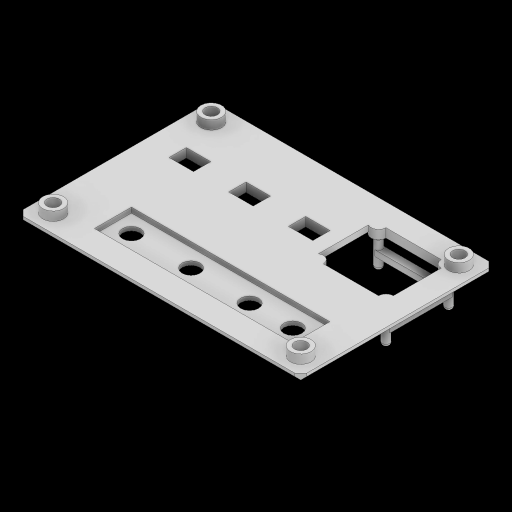
# Autodesk Inventor part: gora
Saved by Autodesk Inventor 2024.4 (Build 284460000, 460)
## iProperties
Created: 2026-01-14
Part Number: gora
Material: Ogólny
Document SubType Name: Modeling
Designer: User
Density: 1 g/cm^3
Appearance: Domyślna
Author: User
Autodesk Inventor part; units mm, degrees
ref_plane "YZ Plane" through (0, 0, 0) normal (1, 0, 0) x (0, 1, 0)
ref_plane "XZ Plane" through (0, 0, 0) normal (0, 1, 0) x (-1, 0, 0)
ref_plane "XY Plane" through (0, 0, 0) normal (0, 0, 1) x (1, 0, 0)
sketch "Szkic1" plane through (0, 0, 0) normal (0, 1, 0) x (-1, 0, 0)
  line L0 (-47.5, 32.5) -> (47.5, 32.5)
  line L1 (47.5, 32.5) -> (47.5, -32.5)
  line L2 (47.5, -32.5) -> (-47.5, -32.5)
  line L3 (-47.5, -32.5) -> (-47.5, 32.5)
  line L4 (-47.5, 32.5) -> (47.5, -32.5) construction
  line L5 (47.5, 32.5) -> (-47.5, -32.5) construction
  point P0 (0, 0)
  dimension "d0" = 95
  dimension "d1" = 65
  constraints: 12 end point, 2 midpoint, 2 parallel, 1 horizontal, 1 perpendicular
  measures "d0" distance of L1.end L2.end
  measures "d1" distance of L0.end L1.end
extrude "Wyciągnięcie proste1" add sketch "Szkic1" along normal blind 3
chamfer "Faza1" distance 2 angle 45 4 edges at (47.5, 1.5, 32.5) (47.5, 1.5, -32.5) (-47.5, 1.5, 32.5) (-47.5, 1.5, -32.5)
sketch "Szkic4" plane through (0, 0, 0) normal (0, -1, 0) x (1, 0, 0)
  line L0 (41.8196, -27.3452) -> (14.8196, -27.3452)
  line L1 (16.8196, -2.3452) -> (41.8196, -2.3452)
  line L2 (15.8196, -27.5) -> (42.8196, -27.5)
  line L3 (41.8196, -2.3452) -> (41.8196, -27.3452)
  line L4 (41.8196, -27.3452) -> (14.8196, -2.3452) construction
  line L5 (14.8196, -27.3452) -> (41.8196, -2.3452) construction
  circle A0 centre (39.5696, -25) radius 1.25
  circle A1 centre (38.3196, -4.5952) radius 1.25
  circle A2 centre (39.5696, -4) radius 1.25
  circle A3 centre (17.3196, -4.5952) radius 1.25
  circle A4 centre (16.0696, -4) radius 1.25
  circle A5 centre (17.3196, -28.0952) radius 1.25
  circle A6 centre (16.0696, -25) radius 1.25
  circle A7 centre (38.3196, -28.0952) radius 1.25
  line L6 (13.8196, -2.3452) -> (13.8196, -28.3452)
  line L7 (12.8196, -1.5) -> (40.8196, -1.5)
  line L8 (41.8196, -28.3452) -> (41.8196, -2.3452)
  line L9 (14.8196, -2.3452) -> (14.8196, -30.3452)
  line L10 (14.8196, -30.3452) -> (40.8196, -2.3452) construction
  line L11 (40.8196, -30.3452) -> (14.8196, -2.3452) construction
  line L12 (34.7997, -21.2897) -> (22.7997, -21.2897)
  line L13 (22.7997, -21.2897) -> (22.7997, -9.2897)
  line L14 (22.7997, -9.2897) -> (34.7997, -9.2897)
  line L15 (34.7997, -9.2897) -> (34.7997, -21.2897)
  line L16 (34.7997, -21.2897) -> (22.7997, -9.2897) construction
  line L17 (22.7997, -21.2897) -> (34.7997, -9.2897) construction
  line L18 (39.5696, -25) -> (16.0696, -25)
  line L19 (16.0696, -25) -> (16.0696, -4)
  line L20 (16.0696, -4) -> (39.5696, -4)
  line L21 (39.5696, -4) -> (39.5696, -25)
  circle A8 centre (16.0696, -25) radius 2.5
  circle A9 centre (39.5696, -25) radius 2.5
  circle A10 centre (39.5696, -4) radius 2.5
  circle A11 centre (16.0696, -4) radius 2.5
  line L22 (45.5, -32.5) -> (-45.5, -32.5) projected
  point P0 (0, 0)
  point P1 (28.3196, -14.8452)
  point P2 (27.8196, -16.3452)
  point P3 (28.7997, -15.2897)
  point P4 (18.5696, -4)
  point P5 (16.0696, -6.5)
  point P6 (16.0696, -22.5)
  point P7 (18.5696, -25)
  point P8 (37.0696, -25)
  point P9 (39.5696, -22.5)
  point P10 (39.5696, -6.5)
  point P11 (37.0696, -4)
  dimension "d36" = 27
  dimension "d37" = 25
  dimension "d41" = 26
  dimension "d42" = 28
  dimension "d43" = 12
  dimension "d44" = 12
  dimension "d62" = 18.5
  dimension "d63" = 5
  dimension "d64" = 5
  dimension "d65" = 5
  dimension "d66" = 5
  dimension "d79" = 7.5
  dimension "d80" = 2.5
  dimension "d81" = 90
  dimension "d82" = 42.797
  dimension "d83" = 137.203
  dimension "d84" = 132.879
  dimension "d85" = 47.121
  dimension "d86" = 90
  dimension "d87" = 5.1548
  dimension "d88" = 23.2103
  dimension "d89" = 28
  dimension "d90" = 4.7699
  dimension "d91" = 23.5
  dimension "d92" = 3.6804
  dimension "d93" = 3.6804
  dimension "d94" = 30.1548
  dimension "d95" = 24.6269
  dimension "d96" = 1.9635
  dimension "d97" = 30.1548
  dimension "d98" = 30.1548
  dimension "d99" = 30.1548
  dimension "d100" = 30.1548
  dimension "d101" = 2.1548
  dimension "d102" = 25.1548
  dimension "d103" = 9.1548
  dimension "d104" = 27.9048
  dimension "d105" = 4.4048
  dimension "d106" = 27.6548
  dimension "d107" = 6.6548
  dimension "d108" = 27.6548
  dimension "d109" = 6.6548
  dimension "d110" = 27.9048
  dimension "d111" = 4.4048
  dimension "d112" = 25.1548
  dimension "d113" = 9.1548
  dimension "d114" = 30.1548
  dimension "d115" = 2.1548
  dimension "d116" = 30.1548
  dimension "d117" = 4.1548
  dimension "d118" = 1
  dimension "d119" = 0
  dimension "d120" = 1
  dimension "d121" = 2.25
  dimension "d122" = 2.25
  dimension "d123" = 4.75
  dimension "d124" = 4.75
  dimension "d125" = 23.25
  dimension "d126" = 23.25
  dimension "d127" = 25.75
  dimension "d128" = 25.75
  dimension "d129" = 27
  constraints: 44 end point, 12 centre point, 9 tangent, 7 parallel, 6 equal radius, 6 midpoint, 4 coincident, 3 horizontal, 3 perpendicular, 2 concentric, 2 point on line
  measures "d36" distance of L2.start L2.end
  measures "d37" distance of L1.start L1.end
  measures "d41" distance of L8.end L8.start
  measures "d42" distance of L7.start L7.end
  measures "d43" distance of L13.end L14.end
  measures "d44" distance of L12.end L13.end
  measures "d63" diameter of A8
  measures "d64" diameter of A9
  measures "d65" diameter of A10
  measures "d66" diameter of A11
  measures "d79" distance between parallel lines of L22 L18
  measures "d80" diameter of A2
  measures "d81" angle of L3 L22
  measures "d82" angle of L4 L22
  measures "d83" angle of L5 L22
  measures "d84" angle of L10 L22
  measures "d85" angle of L11 L22
  measures "d86" angle of L3 L1
  measures "d87" distance between parallel lines of L0 L22
  measures "d88" distance between parallel lines of L14 L22
  measures "d89" distance between parallel lines of L8 L6
  measures "d90" distance between parallel lines of L21 L15
  measures "d91" distance between parallel lines of L21 L19
  measures "d92" distance from line of L22.start L3
  measures "d93" distance from line of L22.start L8
  measures "d94" distance from line of L22.start L1
  measures "d95" distance from line of L22.start L5
  measures "d96" distance from line of L22.start L11
  measures "d97" distance from line of L8.end L22
  measures "d98" distance from line of L3.start L22
  measures "d99" distance from line of L5.end L22
  measures "d100" distance from line of L10.end L22
  measures "d101" distance from line of L11.start L22
  measures "d104" distance from line of A1.centre L22
  measures "d105" distance from line of A7.centre L22
  measures "d110" distance from line of A3.centre L22
  measures "d111" distance from line of A5.centre L22
  measures "d114" distance from line of L9.start L22
  measures "d115" distance from line of L9.end L22
  measures "d116" distance from line of L6.start L22
  measures "d117" distance from line of L6.end L22
  measures "d118" distance from line of L2.end L3
  measures "d119" distance from line of L1.end L3
  measures "d120" distance from line of L7.end L3
  measures "d121" distance from line of point (39.57, -6.5) L3
  measures "d122" distance from line of point (39.57, -22.5) L3
  measures "d123" distance from line of point (37.07, -4) L3
  measures "d124" distance from line of point (37.07, -25) L3
  measures "d125" distance from line of point (18.57, -4) L3
  measures "d126" distance from line of point (18.57, -25) L3
  measures "d127" distance from line of point (16.07, -6.5) L3
  measures "d128" distance from line of point (16.07, -22.5) L3
  measures "d129" distance from line of L0.end L3
extrude "Wyciągnięcie proste6" add sketch "Szkic4" along normal blind 10 contours L21 L18 A0 | A0 L18 L21 | L21 L20 A1 A2 | A2 A1 L21 | L18 L19 A6 | A6 L19 L18 | A2 L20 A1 | A1 L20 L21 | A2 A1 L20 | L19 A3 A4 | A4 A3 L20 L19 | A3 L20 A4 | L19 L20 A3 | A4 L20 A3 picked at (38.7441, -4.2892) picked at (38.9967, -3.9208) picked at (16.8951, -4.2892) picked at (16.6425, -3.9208)
fillet "Zaokrąglenie1" radius 1 4 edges at (14.8196, 0, -4) (14.8196, 0, -25) (38.3196, 0, -25) (38.3196, 0, -4)
sketch "Szkic6" plane through (0, 3, 0) normal (0, 1, 0) x (1, 0, 0)
  line L0 (47.5, -30.5) -> (47.5, 30.5) projected
  line L1 (47.5, 0) -> (-47.5, 0)
  line L2 (-47.5, 30.5) -> (-47.5, -30.5) projected
  line L3 (45.5, 32.5) -> (-45.5, 32.5) projected
  line L4 (0, 32.5) -> (0, -32.5)
  line L5 (-45.5, -32.5) -> (45.5, -32.5) projected
  circle A0 centre (41.5, -26.5) radius 2.1
  circle A1 centre (41.5, -26.5) radius 3.5
  line L6 (41.5, -26.5) -> (41.5, 26.5)
  circle A2 centre (41.5, 26.5) radius 2
  line L7 (41.5, -26.5) -> (-41.5, -26.5)
  line L8 (41.5, -26.5) -> (124.5, -26.5) construction
  circle A3 centre (-41.5, -26.5) radius 2
  point P0 (0, 0)
  dimension "d56" = 6
  dimension "d57" = 6
  dimension "d58" = 7
  dimension "d59" = 4.2
  dimension "d133" = 53
  dimension "d134" = 4
  dimension "d135" = 6
  dimension "d136" = 6
  dimension "d137" = 83
  dimension "d138" = 180
  dimension "d139" = 4
  dimension "d140" = 6
  dimension "d141" = 6
  constraints: 10 end point, 4 centre point, 4 midpoint, 3 coincident, 2 horizontal, 1 collinear, 1 vertical
  measures "d56" distance from line of L0 A0.centre
  measures "d57" distance from line of L5 A0.centre
  measures "d58" diameter of A1
  measures "d59" diameter of A0
  measures "d133" distance of L6.start L6.end
  measures "d134" diameter of A2
  measures "d135" distance from line of L3 A2.centre
  measures "d136" distance from line of L0 A2.centre
  measures "d137" distance of L6.start L7.end
  measures "d138" angle of L7 L8
  measures "d139" diameter of A3
  measures "d140" distance from line of L2 A3.centre
  measures "d141" distance from line of L5 A3.centre
extrude "Wyciągnięcie proste8" add sketch "Szkic6" along normal blind 3 contours L6 A0 L7 A1 | A1 L7 A0 L6
extrude "Wyciągnięcie proste9" cut sketch "Szkic4" against normal blind 4 contours A9 L18 A8 L19 A11 A3 L20 A10 A1 L21 | A1 A10 | A11 A3 | L12 L13 L14 L15
move faces "Przesuń3" translate (-1.25, 0, 0) faces at (16.0696, 1, -11.8333)
ref_plane "Płaszczyzna konstrukcyjna1" through (16.0696, -5, -4) normal (0, -1, 0) x (1, 0, 0)
sketch "Szkic7" plane through (16.0696, -5, -4) normal (0, -1, 0) x (1, 0, 0)
  circle A0 centre (0, 0) radius 1.25 projected
  circle A1 centre (23.5, 0) radius 1.25 projected
  line L0 (0, 1.25) -> (23.5, 1.25)
  line L1 (23.5, 1.25) -> (23.5, -1.25)
  line L2 (23.5, -1.25) -> (0, -1.25)
  line L3 (0, -1.25) -> (0, 1.25)
  circle A2 centre (23.5, -21) radius 1.25 projected
  line L4 (24.75, 0) -> (22.25, 0)
  line L5 (22.25, 0) -> (22.25, -21)
  line L6 (22.25, -21) -> (24.75, -21)
  line L7 (24.75, -21) -> (24.75, 0)
  line L8 (23.5, -22.25) -> (0, -22.25)
  line L9 (0, -22.25) -> (0, -19.75)
  line L10 (0, -19.75) -> (23.5, -19.75)
  line L11 (23.5, -19.75) -> (23.5, -22.25)
  circle A3 centre (0, -21) radius 1.25 projected
  line L12 (-1.25, -21) -> (1.25, -21)
  line L13 (1.25, -21) -> (1.25, 0)
  line L14 (1.25, 0) -> (-1.25, 0)
  line L15 (-1.25, 0) -> (-1.25, -21)
  point P0 (-16.0696, 4)
  point P1 (24.75, -21)
  point P2 (22.25, -1.25)
  point P3 (22.25, -19.75)
  point P4 (1.25, -19.75)
  point P5 (1.25, -1.25)
  constraints: 32 end point, 8 parallel, 7 point on circle, 4 horizontal, 4 perpendicular
extrude "Wyciągnięcie proste10" add sketch "Szkic7" along normal mid plane 2 contours L13 L2 A0 | A0 L0 A1 L5 L2 L13 | L2 A1 L7 A2 L10 L5 | L13 A3 L10 | L10 L5 A2 L8 A3 L13
fillet "Zaokrąglenie2" radius 1 4 edges at (14.8196, -10, -4) (14.8196, -10, -25) (38.3196, -10, -25) (38.3196, -10, -4)
chamfer "Faza2" distance 1 angle 45 1 edges at (14.8196, 0, -14.5)
mirror "Odbij1" about plane through (0, 0, 0) normal (0, 0, 1) of "Wyciągnięcie proste8"
mirror "Odbij2" about plane through (0, 0, 0) normal (1, 0, 0) of "Wyciągnięcie proste8", "Odbij1"
chamfer "Faza3" distance 2 angle 45 4 edges at (0, 0, -32.5) (47.5, 0, 0) (0, 0, 32.5) (-47.5, 0, 0)
sketch "Szkic8" plane through (0, 0, 0) normal (0, -1, 0) x (1, 0, 0)
  point P0 (0, 0)
sketch "Szkic9" plane through (0, 0, 0) normal (0, -1, 0) x (1, 0, 0)
  line L0 (-23.3666, -57.3233) -> (-23.3666, -67.3233)
  line L1 (-23.3666, -67.3233) -> (-33.3666, -67.3233)
  line L2 (-33.3666, -67.3233) -> (-33.3666, -57.3233)
  line L3 (-33.3666, -57.3233) -> (-23.3666, -57.3233)
  circle A0 centre (-28.3666, -62.3233) radius 1.65
  line L4 (-23.3666, -57.3233) -> (-33.3666, -67.3233) construction
  line L5 (-23.3666, -67.3233) -> (-33.3666, -57.3233) construction
  line L6 (-33.3666, -67.3233) -> (-33.3666, -57.3233)
  line L7 (-33.3666, -57.3233) -> (30.5704, -57.3233)
  line L8 (30.5704, -57.3233) -> (30.5704, -67.3233)
  line L9 (30.5704, -67.3233) -> (-33.3666, -67.3233)
  line L10 (-28.3666, -62.3233) -> (-28.3666, -82.3233)
  line L11 (-24.7466, -85.2233) -> (-24.7466, -79.6233)
  line L12 (-24.7466, -79.6233) -> (-31.1466, -79.6233)
  line L13 (-31.1466, -79.6233) -> (-31.1466, -85.2233)
  line L14 (-31.1466, -85.2233) -> (-24.7466, -85.2233)
  line L15 (-24.7466, -85.2233) -> (-31.1466, -79.6233) construction
  line L16 (-24.7466, -79.6233) -> (-31.1466, -85.2233) construction
  line L17 (-4.7466, -79.6233) -> (-11.1466, -79.6233)
  line L18 (-8.3666, -62.3233) -> (-8.3666, -82.3233)
  line L19 (-4.7466, -85.2233) -> (-4.7466, -79.6233)
  line L20 (-11.1466, -79.6233) -> (-11.1466, -85.2233)
  line L21 (-11.1466, -85.2233) -> (-4.7466, -85.2233)
  line L22 (-4.7466, -79.6233) -> (-11.1466, -85.2233) construction
  line L23 (-4.7466, -85.2233) -> (-11.1466, -79.6233) construction
  line L24 (15.2534, -79.6233) -> (8.8534, -79.6233)
  line L25 (11.6334, -62.3233) -> (11.6334, -82.3233)
  line L26 (15.2534, -85.2233) -> (15.2534, -79.6233)
  line L27 (8.8534, -79.6233) -> (8.8534, -85.2233)
  line L28 (8.8534, -85.2233) -> (15.2534, -85.2233)
  line L29 (15.2534, -79.6233) -> (8.8534, -85.2233) construction
  line L30 (15.2534, -85.2233) -> (8.8534, -79.6233) construction
  line L31 (-45.5, 30.5) -> (45.5, 30.5) projected
  line L32 (0, 30.5) -> (0, 17.7)
  line L33 (30.5, 20.7) -> (-30.5, 20.7)
  line L34 (-30.5, 20.7) -> (-30.5, 14.7)
  line L35 (-30.5, 14.7) -> (30.5, 14.7)
  line L36 (30.5, 14.7) -> (30.5, 20.7)
  line L37 (30.5, 20.7) -> (-30.5, 14.7) construction
  line L38 (-30.5, 20.7) -> (30.5, 14.7) construction
  line L39 (-30.5, 17.7) -> (-24.05, 17.7)
  circle A1 centre (-24.05, 17.7) radius 3
  circle A2 centre (-4.05, 17.7) radius 3
  circle A3 centre (15.95, 17.7) radius 3
  circle A4 centre (30.45, 17.7) radius 3
  point P0 (0, 0)
  point P1 (73.1005, -3.8431)
  point P2 (-27.9466, -82.4233)
  point P3 (-7.9466, -82.4233)
  point P4 (12.0534, -82.4233)
  dimension "d146" = 10
  dimension "d147" = 10
  dimension "d148" = 10
  dimension "d149" = 20
  dimension "d150" = 5.6
  dimension "d151" = 6.4
  dimension "d152" = 20
  dimension "d153" = 17.9
  dimension "d154" = 3.62
  dimension "d155" = 55.317
  dimension "d157" = 12.8
  dimension "d158" = 61
  dimension "d159" = 6
  dimension "d160" = 6.45
  dimension "d161" = 6
  dimension "d166" = 20
  dimension "d173" = 14.5
  constraints: 78 end point, 8 midpoint, 8 parallel, 5 centre point, 5 horizontal, 4 perpendicular, 1 coincident, 1 vertical, 34 other
  measures "d146" distance of L1.end L2.end
  measures "d147" distance of L0.end L1.end
  measures "d148" distance of L7.end L8.end
  measures "d149" distance of L10.start L10.end
  measures "d150" distance of L13.end L12.end
  measures "d151" distance of L12.end L11.end
  measures "d152" distance of L10.end L18.end
  measures "d153" distance between parallel lines of L14 L1
  measures "d154" distance between parallel lines of L10 L11
  measures "d155" distance between parallel lines of L8 L11
  measures "d157" distance of L32.start L32.end
  measures "d158" distance of L35.end L34.end
  measures "d159" distance of L34.end L33.end
  measures "d160" distance of L39.start L39.end
  measures "d161" diameter of A1
  measures "d166" distance of A1.centre A2.centre
  measures "d173" distance of A3.centre A4.centre
extrude "Wyciągnięcie proste11" cut sketch "Szkic9" against normal blind 3 contours A4 L36 | L36 A4 | A3 | A2 | A1
move faces "Przesuń4" translate (0, 0, 0.4) faces at (18.9403, 2, 17.4586) (33.4403, 2, 17.4586)
ref_plane "Płaszczyzna konstrukcyjna3" through (0, 6.5, 0) normal (0, -1, 0) x (1, 0, 0)
sketch "Szkic10" plane through (0, 6.5, 0) normal (0, -1, 0) x (1, 0, 0)
  line L0 (-18.05, 11.7) -> (-30.05, 11.7)
  line L1 (-30.05, 11.7) -> (-30.05, 23.7)
  line L2 (-30.05, 23.7) -> (-18.05, 23.7)
  line L3 (-18.05, 23.7) -> (-18.05, 11.7)
  circle A0 centre (-24.05, 17.7) radius 3 projected
  line L4 (-18.05, 11.7) -> (-30.05, 23.7) construction
  line L5 (-30.05, 11.7) -> (-18.05, 23.7) construction
  line L6 (36.45, 12.1) -> (24.45, 12.1)
  line L7 (24.45, 12.1) -> (24.45, 24.1)
  line L8 (24.45, 24.1) -> (36.45, 24.1)
  line L9 (36.45, 24.1) -> (36.45, 12.1)
  circle A1 centre (30.45, 18.1) radius 3 projected
  line L10 (36.45, 12.1) -> (24.45, 24.1) construction
  line L11 (24.45, 12.1) -> (36.45, 24.1) construction
  line L12 (-30.05, 11.7) -> (36.45, 11.7)
  line L13 (36.45, 11.7) -> (36.45, 24.1)
  line L14 (36.45, 24.1) -> (-30.05, 24.1)
  line L15 (-30.05, 24.1) -> (-30.05, 11.7)
  point P0 (0, 0)
  dimension "d182" = 12
  dimension "d183" = 12
  dimension "d184" = 12
  dimension "d185" = 12
  constraints: 32 end point, 6 parallel, 4 midpoint, 3 horizontal, 3 perpendicular
  measures "d182" distance of L1.end L2.end
  measures "d183" distance of L0.end L1.end
  measures "d184" distance of L7.end L8.end
  measures "d185" distance of L6.end L7.end
extrude "Wyciągnięcie proste12" cut sketch "Szkic10" along normal blind 5.2
sketch "Szkic11" plane through (0, 0, 0) normal (0, -1, 0) x (1, 0, 0)
  circle A0 centre (15.95, 18.1) radius 3 projected
  line L0 (15.95, 18.1) -> (15.95, -11.9)
  line L1 (15.95, -11.9) -> (5.95, -11.9)
  line L2 (10.05, -14.8) -> (1.85, -14.8)
  line L3 (1.85, -14.8) -> (1.85, -9)
  line L4 (1.85, -9) -> (10.05, -9)
  line L5 (10.05, -9) -> (10.05, -14.8)
  line L6 (10.05, -14.8) -> (1.85, -9) construction
  line L7 (1.85, -14.8) -> (10.05, -9) construction
  line L8 (-18.15, -9) -> (-9.95, -9)
  line L9 (-9.95, -9) -> (-9.95, -14.8)
  line L10 (-9.95, -14.8) -> (-18.15, -14.8)
  line L11 (-18.15, -14.8) -> (-18.15, -9)
  line L12 (-38.15, -9) -> (-29.95, -9)
  line L13 (-29.95, -9) -> (-29.95, -14.8)
  line L14 (-29.95, -14.8) -> (-38.15, -14.8)
  line L15 (-38.15, -14.8) -> (-38.15, -9)
  point P0 (0, 0)
  dimension "d188" = 30
  dimension "d189" = 10
  dimension "d190" = 8.2
  dimension "d191" = 5.8
  dimension "d194" = 20
  constraints: 32 end point, 2 horizontal, 2 midpoint, 2 parallel, 2 perpendicular, 1 vertical, 16 other
  measures "d188" distance of L0.start L0.end
  measures "d189" distance of L0.end L1.end
  measures "d190" distance of L3.end L4.end
  measures "d191" distance of L2.end L3.end
  measures "d194" distance of L3.end L8.start
extrude "Wyciągnięcie proste13" cut sketch "Szkic11" against normal blind 7.45 contours L2 L3 L4 L5 | L8 L9 L10 L11 | L12 L13 L14 L15
sketch "Szkic12" plane through (0, 0, 0) normal (0, -1, 0) x (1, 0, 0)
  line L0 (-36.4487, 3.4721) -> (-36.4487, 10.2829) construction
  line L1 (-36.4487, 10.2829) -> (-27.9352, 10.2829) construction
  line L2 (-27.9352, 10.2829) -> (-27.9352, 3.4721) construction
  line L3 (-27.9352, 3.4721) -> (-36.4487, 3.4721) construction
  line L4 (-34.05, -8.1767) -> (-38.2926, -3.9341)
  line L5 (-34.05, -8.1767) -> (-28.05, -8.1767) construction
  line L6 (-34.05, -8.1767) -> (-29.8074, -3.9341)
  line L7 (-29.8074, -3.9341) -> (-32.8074, -3.9341)
  line L8 (-38.2926, -3.9341) -> (-35.2926, -3.9341)
  line L9 (-24.0069, 13.77) -> (-19.7643, 9.5273)
  line L10 (-24.0069, 13.77) -> (-18.0069, 13.77) construction
  line L11 (-24.0069, 13.77) -> (-28.2496, 9.5273)
  line L12 (-28.2496, 9.5273) -> (-25.2496, 9.5273)
  line L13 (-19.7643, 9.5273) -> (-22.7643, 9.5273)
  line L14 (-22.7643, 9.5273) -> (-22.7643, 4.5273)
  line L15 (-32.8074, -3.9341) -> (-32.8074, 1.0659)
  line L16 (-32.8074, 1.0659) -> (-22.7643, 1.0659)
  line L17 (-22.7643, 1.0659) -> (-22.7643, 4.5273)
  line L18 (-35.2926, -3.9341) -> (-35.2926, 2.4842)
  line L19 (-35.2926, 2.4842) -> (-35.2926, 3.5509)
  line L20 (-35.2926, 3.5509) -> (-25.2496, 3.5509)
  line L21 (-25.2496, 3.5509) -> (-25.2496, 9.5273)
  line L22 (-15.2926, 2.4842) -> (-15.2926, 3.5509)
  line L23 (-15.2926, 3.5509) -> (-5.2496, 3.5509)
  line L24 (-12.8074, 1.0659) -> (-2.7643, 1.0659)
  line L25 (-2.7643, 1.0659) -> (-2.7643, 4.5273)
  line L26 (-5.2496, 3.5509) -> (-5.2496, 9.5273)
  line L27 (-8.2496, 9.5273) -> (-5.2496, 9.5273)
  line L28 (-2.7643, 9.5273) -> (-2.7643, 4.5273)
  line L29 (-4.0069, 13.77) -> (-8.2496, 9.5273)
  line L30 (0.2357, 9.5273) -> (-2.7643, 9.5273)
  line L31 (-4.0069, 13.77) -> (0.2357, 9.5273)
  line L32 (-4.0069, 13.77) -> (1.9931, 13.77) construction
  line L33 (-15.2926, -3.9341) -> (-15.2926, 2.4842)
  line L34 (-12.8074, -3.9341) -> (-12.8074, 1.0659)
  line L35 (-9.8074, -3.9341) -> (-12.8074, -3.9341)
  line L36 (-18.2926, -3.9341) -> (-15.2926, -3.9341)
  line L37 (-14.05, -8.1767) -> (-8.05, -8.1767) construction
  line L38 (-14.05, -8.1767) -> (-9.8074, -3.9341)
  line L39 (-14.05, -8.1767) -> (-18.2926, -3.9341)
  line L40 (4.7074, 2.4842) -> (4.7074, 3.5509)
  line L41 (4.7074, 3.5509) -> (14.7504, 3.5509)
  line L42 (7.1926, 1.0659) -> (17.2357, 1.0659)
  line L43 (17.2357, 1.0659) -> (17.2357, 4.5273)
  line L44 (14.7504, 3.5509) -> (14.7504, 9.5273)
  line L45 (11.7504, 9.5273) -> (14.7504, 9.5273)
  line L46 (17.2357, 9.5273) -> (17.2357, 4.5273)
  line L47 (15.9931, 13.77) -> (11.7504, 9.5273)
  line L48 (20.2357, 9.5273) -> (17.2357, 9.5273)
  line L49 (15.9931, 13.77) -> (20.2357, 9.5273)
  line L50 (15.9931, 13.77) -> (21.9931, 13.77) construction
  line L51 (4.7074, -3.9341) -> (4.7074, 2.4842)
  line L52 (7.1926, -3.9341) -> (7.1926, 1.0659)
  line L53 (10.1926, -3.9341) -> (7.1926, -3.9341)
  line L54 (1.7074, -3.9341) -> (4.7074, -3.9341)
  line L55 (5.95, -8.1767) -> (11.95, -8.1767) construction
  line L56 (5.95, -8.1767) -> (10.1926, -3.9341)
  line L57 (5.95, -8.1767) -> (1.7074, -3.9341)
  line L58 (-16.1178, 3.1562) -> (-16.1178, 9.967) construction
  line L59 (-16.1178, 9.967) -> (-7.6042, 9.967) construction
  line L60 (-7.6042, 9.967) -> (-7.6042, 3.1562) construction
  line L61 (-7.6042, 3.1562) -> (-16.1178, 3.1562) construction
  line L62 (3.3746, 3.2527) -> (3.3746, 10.0635) construction
  line L63 (3.3746, 10.0635) -> (11.8881, 10.0635) construction
  line L64 (11.8881, 10.0635) -> (11.8881, 3.2527) construction
  line L65 (11.8881, 3.2527) -> (3.3746, 3.2527) construction
  line L66 (42.8638, 11.2188) -> (34.3502, 11.2188) construction
  line L67 (34.3502, 11.2188) -> (34.3502, 18.0296) construction
  line L68 (34.3502, 18.0296) -> (42.8638, 18.0296) construction
  line L69 (42.8638, 18.0296) -> (42.8638, 11.2188) construction
  line L70 (-29.692, 8.7637) -> (-29.692, 5.429)
  line L71 (-29.692, 5.429) -> (-34.692, 5.429)
  line L72 (-34.692, 5.429) -> (-34.692, 6.6851)
  line L73 (-34.692, 6.6851) -> (-30.6442, 6.6851)
  line L74 (-30.6442, 6.6851) -> (-30.6442, 8.7637)
  line L75 (-30.6442, 8.7637) -> (-29.692, 8.7637)
  line L76 (-9.361, 9.2034) -> (-9.361, 7.6758)
  line L77 (-9.361, 7.6758) -> (-11.1965, 6.286)
  line L78 (-11.1965, 6.286) -> (-11.1965, 5.8322)
  line L79 (-11.1965, 5.8322) -> (-9.361, 5.8322)
  line L80 (-9.361, 5.8322) -> (-9.361, 4.5843)
  line L81 (-9.361, 4.5843) -> (-14.361, 4.5843)
  line L82 (-14.361, 4.5843) -> (-14.361, 6.594)
  spline S0 degree 2 poles (-14.361, 6.594) (-14.361, 7.0113) (-14.2557, 7.6272) (-14.0936, 7.8906) knots 0 0 0 1 2 2 2
  spline S1 degree 2 poles (-14.0936, 7.8906) (-13.9234, 8.158) (-13.3926, 8.4741) (-12.9874, 8.4741) knots 0 0 0 1 2 2 2
  spline S2 degree 2 poles (-12.9874, 8.4741) (-12.4161, 8.4741) (-11.6989, 7.9554) (-11.4882, 7.5219) knots 0 0 0 1 2 2 2
  line L83 (-11.4882, 7.5219) -> (-9.361, 9.2034)
  spline S3 degree 2 poles (-12.8294, 7.1856) (-13.0198, 7.1856) (-13.2913, 7.0397) (-13.3642, 6.8736) knots 0 0 0 1 2 2 2
  spline S4 degree 2 poles (-13.3642, 6.8736) (-13.4129, 6.7561) (-13.4412, 6.4684) (-13.4412, 6.2536) knots 0 0 0 1 2 2 2
  line L84 (-13.4412, 6.2536) -> (-13.4412, 5.8322)
  line L85 (-13.4412, 5.8322) -> (-12.096, 5.8322)
  line L86 (-12.096, 5.8322) -> (-12.096, 6.1929)
  spline S5 degree 2 poles (-12.096, 6.1929) (-12.096, 6.4522) (-12.1608, 6.8209) (-12.2621, 6.9465) knots 0 0 0 1 2 2 2
  spline S6 degree 2 poles (-12.2621, 6.9465) (-12.3594, 7.0681) (-12.6187, 7.1856) (-12.8294, 7.1856) knots 0 0 0 1 2 2 2
  spline S7 degree 2 poles (10.2286, 7.0369) (10.2286, 5.9105) (8.8671, 4.5896) (7.6354, 4.5896) knots 0 0 0 1 2 2 2
  spline S8 degree 2 poles (7.6354, 4.5896) (6.4482, 4.5896) (5.0341, 5.9146) (5.0341, 7.041) knots 0 0 0 1 2 2 2
  spline S9 degree 2 poles (5.0341, 7.041) (5.0341, 7.3368) (5.1029, 7.8149) (5.1597, 8.0337) knots 0 0 0 1 2 2 2
  spline S10 degree 2 poles (5.1597, 8.0337) (5.2124, 8.2039) (5.3866, 8.605) (5.4514, 8.7306) knots 0 0 0 1 2 2 2
  line L87 (5.4514, 8.7306) -> (6.6427, 8.7306)
  line L88 (6.6427, 8.7306) -> (6.6427, 8.605)
  spline S11 degree 2 poles (6.6427, 8.605) (6.5616, 8.5118) (6.3347, 8.2363) (6.2294, 8.062) knots 0 0 0 1 2 2 2
  spline S12 degree 2 poles (6.2294, 8.062) (6.12, 7.8878) (5.97, 7.4705) (5.97, 7.2395) knots 0 0 0 1 2 2 2
  spline S13 degree 2 poles (5.97, 7.2395) (5.97, 6.968) (6.1402, 6.5183) (6.355, 6.3116) knots 0 0 0 1 2 2 2
  spline S14 degree 2 poles (6.355, 6.3116) (6.5454, 6.1252) (7.1978, 5.8862) (7.6394, 5.8862) knots 0 0 0 1 2 2 2
  spline S15 degree 2 poles (7.6394, 5.8862) (8.1054, 5.8862) (8.7415, 6.1334) (8.936, 6.3359) knots 0 0 0 1 2 2 2
  spline S16 degree 2 poles (8.936, 6.3359) (9.1265, 6.5304) (9.2926, 7.0086) (9.2926, 7.2476) knots 0 0 0 1 2 2 2
  spline S17 degree 2 poles (9.2926, 7.2476) (9.2926, 7.4948) (9.1265, 7.9445) (9.0252, 8.0985) knots 0 0 0 1 2 2 2
  spline S18 degree 2 poles (9.0252, 8.0985) (8.9239, 8.2687) (8.7091, 8.524) (8.624, 8.6171) knots 0 0 0 1 2 2 2
  line L89 (8.624, 8.6171) -> (8.624, 8.7306)
  line L90 (8.624, 8.7306) -> (9.7991, 8.7306)
  spline S19 degree 2 poles (9.7991, 8.7306) (9.8639, 8.5928) (10.026, 8.2322) (10.0827, 8.0377) knots 0 0 0 1 2 2 2
  spline S20 degree 2 poles (10.0827, 8.0377) (10.1556, 7.8027) (10.2286, 7.3935) (10.2286, 7.0369) knots 0 0 0 1 2 2 2
  spline S21 degree 2 poles (41.1961, 5.4467) (41.1961, 4.8713) (40.9733, 4.0042) (40.8112, 3.6315) knots 0 0 0 1 2 2 2
  line L91 (40.8112, 3.6315) -> (39.62, 3.6315)
  line L92 (39.62, 3.6315) -> (39.62, 3.7449)
  spline S22 degree 2 poles (39.62, 3.7449) (39.9401, 4.1217) (40.2845, 5.0253) (40.2845, 5.4508) knots 0 0 0 1 2 2 2
  spline S23 degree 2 poles (40.2845, 5.4508) (40.2845, 5.5602) (40.2359, 5.9127) (40.1872, 6.018) knots 0 0 0 1 2 2 2
  spline S24 degree 2 poles (40.1872, 6.018) (40.1305, 6.1477) (39.9239, 6.33) (39.7577, 6.33) knots 0 0 0 1 2 2 2
  spline S25 degree 2 poles (39.7577, 6.33) (39.5673, 6.33) (39.3323, 6.0342) (39.2796, 5.8316) knots 0 0 0 1 2 2 2
  spline S26 degree 2 poles (39.2796, 5.8316) (39.2107, 5.5764) (39.0932, 4.997) (39.0041, 4.7417) knots 0 0 0 1 2 2 2
  spline S27 degree 2 poles (39.0041, 4.7417) (38.8015, 4.1623) (38.1086, 3.6598) (37.59, 3.6598) knots 0 0 0 1 2 2 2
  spline S28 degree 2 poles (37.59, 3.6598) (36.889, 3.6598) (36.0179, 4.847) (36.0179, 5.7384) knots 0 0 0 1 2 2 2
  spline S29 degree 2 poles (36.0179, 5.7384) (36.0179, 6.1841) (36.2002, 7.0675) (36.3542, 7.4159) knots 0 0 0 1 2 2 2
  line L93 (36.3542, 7.4159) -> (37.4968, 7.4159)
  line L94 (37.4968, 7.4159) -> (37.4968, 7.3065)
  spline S30 degree 2 poles (37.4968, 7.3065) (37.2577, 7.0269) (36.9295, 6.2247) (36.9295, 5.8033) knots 0 0 0 1 2 2 2
  spline S31 degree 2 poles (36.9295, 5.8033) (36.9295, 5.6371) (36.9782, 5.3778) (37.043, 5.232) knots 0 0 0 1 2 2 2
  spline S32 degree 2 poles (37.043, 5.232) (37.0957, 5.1145) (37.3064, 4.9443) (37.436, 4.9443) knots 0 0 0 1 2 2 2
  spline S33 degree 2 poles (37.436, 4.9443) (37.6305, 4.9443) (37.8534, 5.2158) (37.9425, 5.6047) knots 0 0 0 1 2 2 2
  spline S34 degree 2 poles (37.9425, 5.6047) (37.9992, 5.8559) (38.1086, 6.3219) (38.2018, 6.5893) knots 0 0 0 1 2 2 2
  spline S35 degree 2 poles (38.2018, 6.5893) (38.3923, 7.108) (39.0243, 7.6145) (39.543, 7.6145) knots 0 0 0 1 2 2 2
  spline S36 degree 2 poles (39.543, 7.6145) (40.2885, 7.6145) (41.1961, 6.4435) (41.1961, 5.4467) knots 0 0 0 1 2 2 2
  line L95 (41.107, 9.219) -> (37.0592, 9.219)
  line L96 (37.0592, 9.219) -> (37.0592, 7.7401)
  line L97 (37.0592, 7.7401) -> (36.107, 7.7401)
  line L98 (36.107, 7.7401) -> (36.107, 11.954)
  line L99 (36.107, 11.954) -> (37.0592, 11.954)
  line L100 (37.0592, 11.954) -> (37.0592, 10.4751)
  line L101 (37.0592, 10.4751) -> (41.107, 10.4751)
  line L102 (41.107, 10.4751) -> (41.107, 9.219)
  line L103 (41.107, 11.9297) -> (36.107, 13.6193)
  line L104 (36.107, 13.6193) -> (36.107, 14.9888)
  line L105 (36.107, 14.9888) -> (41.107, 16.6785)
  line L106 (41.107, 16.6785) -> (41.107, 15.3859)
  line L107 (41.107, 15.3859) -> (40.0859, 15.0739)
  line L108 (40.0859, 15.0739) -> (40.0859, 13.5018)
  line L109 (40.0859, 13.5018) -> (41.107, 13.1858)
  line L110 (41.107, 13.1858) -> (41.107, 11.9297)
  line L111 (39.1783, 14.7984) -> (37.5252, 14.2879)
  line L112 (37.5252, 14.2879) -> (39.1783, 13.7733)
  line L113 (39.1783, 13.7733) -> (39.1783, 14.7984)
  line L114 (41.107, 21.796) -> (41.107, 20.2684)
  line L115 (41.107, 20.2684) -> (39.2715, 18.8786)
  line L116 (39.2715, 18.8786) -> (39.2715, 18.4248)
  line L117 (39.2715, 18.4248) -> (41.107, 18.4248)
  line L118 (41.107, 18.4248) -> (41.107, 17.1769)
  line L119 (41.107, 17.1769) -> (36.107, 17.1769)
  line L120 (36.107, 17.1769) -> (36.107, 19.1866)
  spline S37 degree 2 poles (36.107, 19.1866) (36.107, 19.6039) (36.2124, 20.2198) (36.3744, 20.4832) knots 0 0 0 1 2 2 2
  spline S38 degree 2 poles (36.3744, 20.4832) (36.5446, 20.7506) (37.0754, 21.0666) (37.4806, 21.0666) knots 0 0 0 1 2 2 2
  spline S39 degree 2 poles (37.4806, 21.0666) (38.0519, 21.0666) (38.7691, 20.548) (38.9798, 20.1145) knots 0 0 0 1 2 2 2
  line L121 (38.9798, 20.1145) -> (41.107, 21.796)
  spline S40 degree 2 poles (37.6386, 19.7781) (37.4482, 19.7781) (37.1767, 19.6323) (37.1038, 19.4662) knots 0 0 0 1 2 2 2
  spline S41 degree 2 poles (37.1038, 19.4662) (37.0551, 19.3487) (37.0268, 19.061) (37.0268, 18.8462) knots 0 0 0 1 2 2 2
  line L122 (37.0268, 18.8462) -> (37.0268, 18.4248)
  line L123 (37.0268, 18.4248) -> (38.372, 18.4248)
  line L124 (38.372, 18.4248) -> (38.372, 18.7854)
  spline S42 degree 2 poles (38.372, 18.7854) (38.372, 19.0448) (38.3072, 19.4135) (38.2059, 19.5391) knots 0 0 0 1 2 2 2
  spline S43 degree 2 poles (38.2059, 19.5391) (38.1086, 19.6606) (37.8493, 19.7781) (37.6386, 19.7781) knots 0 0 0 1 2 2 2
  line L125 (41.107, 23.129) -> (37.0592, 23.129)
  line L126 (37.0592, 23.129) -> (37.0592, 21.6501)
  line L127 (37.0592, 21.6501) -> (36.107, 21.6501)
  line L128 (36.107, 21.6501) -> (36.107, 25.864)
  line L129 (36.107, 25.864) -> (37.0592, 25.864)
  line L130 (37.0592, 25.864) -> (37.0592, 24.3851)
  line L131 (37.0592, 24.3851) -> (41.107, 24.3851)
  line L132 (41.107, 24.3851) -> (41.107, 23.129)
  point P0 (0, 0)
  dimension "d201" = 6
  dimension "d202" = 135
  dimension "d203" = 6
  dimension "d204" = 3
  dimension "d205" = 3
  dimension "d206" = 90
  dimension "d207" = 6
  dimension "d208" = 315
  dimension "d209" = 6
  dimension "d210" = 3
  dimension "d211" = 3
  dimension "d212" = 90
  dimension "d213" = 5
  dimension "d214" = 5
  dimension "d220" = 20
  constraints: 108 end point, 5 horizontal, 5 vertical, 2 equal length, 2 perpendicular, 1 collinear, 81 other
  measures "d201" distance of L4.start L4.end
  measures "d202" angle of L5 L4
  measures "d203" distance of L4.start L6.end
  measures "d204" distance of L6.end L7.end
  measures "d205" distance of L4.end L8.end
  measures "d206" angle of L4 L6
  measures "d207" distance of L9.start L9.end
  measures "d209" distance of L9.start L11.end
  measures "d210" distance of L11.end L12.end
  measures "d211" distance of L9.end L13.end
  measures "d212" angle of L9 L11
  measures "d213" distance of L13.end L14.end
  measures "d214" distance of L7.end L15.end
  measures "d220" distance of L18.end L22.start
extrude "Wyciągnięcie proste14" cut sketch "Szkic12" against normal blind 0.4
